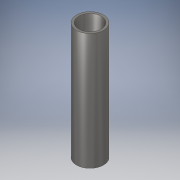
# Autodesk Inventor part: steering_kingpin_bearing_spacer
Saved by Autodesk Inventor 2019 (Build 230136000, 136)
## iProperties
Created: 2019-04-24
Part Number: steering_kingpin_bearing_spacer
Material: Steel, Mild
Document SubType Name: Modeling
Designer: callum.snowden
Mass: 14.1064 g
Surface Area: 36.631 cm^2
Volume: 1.79699 cm^3
Density: 7.85 g/cm^3
Appearance: Semi-Polished
Author: callum.snowden
Autodesk Inventor part; units mm, degrees
ref_plane "YZ Plane" through (0, 0, 0) normal (1, 0, 0) x (0, 1, 0)
ref_plane "XZ Plane" through (0, 0, 0) normal (0, 1, 0) x (-1, 0, 0)
ref_plane "XY Plane" through (0, 0, 0) normal (0, 0, 1) x (1, 0, 0)
sketch "Sketch1" plane through (0, 0, 0) normal (0, 1, 0) x (-1, 0, 0)
  line L0 (0, -8.4) -> (0, 8.4) construction
  line L1 (-8.4, 0) -> (8.4, 0) construction
  circle A0 centre (0, 0) radius 6
  circle A1 centre (0, 0) radius 5
  dimension "d0" = 12
  dimension "d1" = 10
  constraints: 2 centre point, 2 coincident
  measures "d0" diameter of A0
  measures "d1" diameter of A1
extrude "Extrusion1" add sketch "Sketch1" along normal blind 52
body "Solid1"
